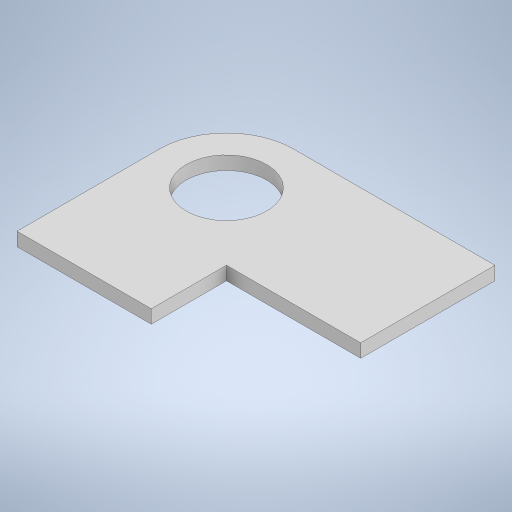
# Autodesk Inventor part: apeature aligner mount
Saved by Autodesk Inventor 2024 (Build 280153000, 153)
## iProperties
Created: 2024-11-08
Part Number: apeature aligner mount
Material: Generic
Document SubType Name: Modeling
Designer: Williamow
Density: 1 g/cm^3
Appearance: Default
Author: Williamow
Autodesk Inventor part; units mm, degrees
ref_plane "YZ Plane" through (0, 0, 0) normal (1, 0, 0) x (0, 1, 0)
ref_plane "XZ Plane" through (0, 0, 0) normal (0, 1, 0) x (-1, 0, 0)
ref_plane "XY Plane" through (0, 0, 0) normal (0, 0, 1) x (1, 0, 0)
sketch "Sketch1" plane through (0, 0, 0) normal (0, 1, 0) x (-1, 0, 0)
  circle A0 centre (0, 0) radius 1.5
  circle A1 centre (0, 0) radius 2.5
  line L0 (2.5, 0) -> (2.5, 5.3)
  line L1 (2.5, 5.3) -> (-2.5, 5.3)
  line L2 (-2.5, 5.3) -> (-2.5, 2.5)
  line L3 (-2.5, 2.5) -> (-7.5, 2.5)
  line L4 (-7.5, 2.5) -> (-7.5, -2.5)
  line L5 (-7.5, -2.5) -> (0, -2.5)
  dimension "d0" = 3
  dimension "d1" = 5
  dimension "d2" = 7.5
  dimension "d3" = 5.3
  constraints: 12 end point, 4 perpendicular, 4 tangent, 2 centre point, 2 coincident, 2 point on circle, 1 horizontal, 1 vertical
  measures "d0" diameter of A0
  measures "d1" diameter of A1
  measures "d2" distance from line of L4 point (0, 0)
  measures "d3" distance from line of L1 point (0, 0)
extrude "Extrusion1" add sketch "Sketch1" along normal blind 0.5
body "Solid1"
